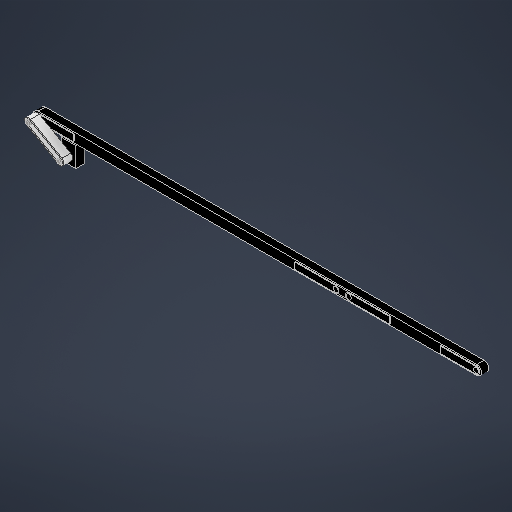
# Autodesk Inventor part: SACMI DPA MAIN CONVEYOR
Saved by Autodesk Inventor 2025 (Build 290162000, 162)
## iProperties
Created: 2024-05-26
Part Number: SACMI DPA MAIN CONVEYOR
Material: Generic
Document SubType Name: Modeling
Designer: zulet
Density: 1 g/cm^3
Appearance: Default
Author: zulet
Autodesk Inventor part; units mm, degrees
ref_plane "YZ Plane" through (0, 0, 0) normal (1, 0, 0) x (0, 1, 0)
ref_plane "XZ Plane" through (0, 0, 0) normal (0, 1, 0) x (-1, 0, 0)
ref_plane "XY Plane" through (0, 0, 0) normal (0, 0, 1) x (1, 0, 0)
sketch "Sketch1" plane through (0, 0, 0) normal (0, 0, 1) x (1, 0, 0)
  line L0 (-1550, 0) -> (1550, 0) construction
  line L1 (-1517, -33) -> (1517, -33)
  line L2 (1517, 33) -> (-1517, 33)
  arc A0 (-1517, 33) -> (-1517, -33) centre (-1517, 0) ccw
  arc A1 (1517, -33) -> (1517, 33) centre (1517, 0) ccw
  line L3 (-1517, 23) -> (1517, 23)
  arc A2 (1517, -23) -> (1517, 23) centre (1517, 0) ccw
  line L4 (1517, -23) -> (-1517, -23)
  arc A3 (-1517, 23) -> (-1517, -23) centre (-1517, 0) ccw
  line L5 (-1268, 23) -> (-1268, -23)
  line L6 (1268, 23) -> (1268, -23)
  circle A4 centre (1517, 0) radius 17.5
  circle A5 centre (-1517, 0) radius 17.5
  arc A6 (523, 0) -> (546, -23) centre (546, 0) ccw construction
  arc A7 (636, 23) -> (636, -23) centre (636, 0) ccw
  line L7 (264, 23) -> (264, -23)
  line L8 (918, 23) -> (918, -23)
  arc A8 (546, 23) -> (523, 0) centre (546, 0) ccw construction
  arc A9 (546, -23) -> (546, 23) centre (546, 0) ccw
  arc A10 (659, 0) -> (636, 23) centre (636, 0) ccw construction
  arc A11 (636, -23) -> (659, 0) centre (636, 0) ccw construction
  circle A12 centre (546, 0) radius 18
  circle A13 centre (636, 0) radius 18
  point P0 (0, 0)
  point P1 (0, 0)
  point P2 (-1550, 0)
  point P3 (1550, 0)
  dimension "d0" = 3100
  dimension "d1" = 66
  dimension "d2" = 10
  dimension "d3" = 282
  dimension "d4" = 282
  dimension "d5" = 35
  dimension "d6" = 35
  dimension "d7" = 282
  dimension "d8" = 282
  dimension "d9" = 90
  dimension "d10" = 350
  dimension "d45" = 5
  dimension "d46" = 5
  constraints: 24 point on circle, 20 end point, 18 point on line, 14 centre point, 8 tangent, 5 coincident, 4 perpendicular, 2 parallel, 1 horizontal, 1 midpoint, 3 other
  measures "d0" distance of L0.start L0.end
  measures "d1" diameter of A1
  measures "d2" distance between parallel lines of L2 L3
  measures "d3" distance from line of point (-1550, 0) L5
  measures "d4" distance from line of point (1550, 0) L6
  measures "d5" diameter of A4
  measures "d6" diameter of A5
  measures "d7" distance from line of L7 A6.centre
  measures "d8" distance from line of L8 A7.centre
  measures "d9" distance of A6.centre A7.centre
  measures "d10" distance between parallel lines of L6 L8
  measures "d45" radial gap between concentric circles of A9 A12
  measures "d46" radial gap between concentric circles of A13 A7
extrude "Extrusion1" add sketch "Sketch1" along normal mid plane 50 contours A0 L2 A1 L1
extrude "Extrusion2" add sketch "Sketch1" along normal mid plane 60 contours L3 L5 L4 A3 | L3 A9 L4 L7 | L3 L8 L4 A7 | L3 A2 L4 L6
extrude "Extrusion3" add sketch "Sketch1" along normal mid plane 50 contours L3 L7 L4 L5 | L3 L6 L4 L8
sketch "Sketch2" plane through (0, 0, 30) normal (0, 0, 1) x (1, 0, 0)
  circle A0 centre (-1517, 0) radius 17.5 projected
  line L0 (-1517, 0) -> (-1300.4936, -125) construction
  line L1 (-1530.75, -23.8157) -> (-1314.2436, -148.8157)
  line L2 (-1286.7436, -101.1843) -> (-1503.25, 23.8157)
  arc A1 (-1503.25, 23.8157) -> (-1530.75, -23.8157) centre (-1517, 0) ccw
  arc A2 (-1314.2436, -148.8157) -> (-1286.7436, -101.1843) centre (-1300.4936, -125) ccw
  line L3 (-1508.25, 15.1554) -> (-1291.7436, -109.8446)
  arc A3 (-1309.2436, -140.1554) -> (-1291.7436, -109.8446) centre (-1300.4936, -125) ccw
  line L4 (-1309.2436, -140.1554) -> (-1525.75, -15.1554)
  arc A4 (-1508.25, 15.1554) -> (-1525.75, -15.1554) centre (-1517, 0) ccw
  line L5 (-1517, -33) -> (1517, -33) projected
  line L6 (-1350.4936, -33) -> (-1250.4936, -33)
  line L7 (-1250.4936, -33) -> (-1250.4936, -175)
  line L8 (-1250.4936, -175) -> (-1350.4936, -175)
  line L9 (-1350.4936, -175) -> (-1350.4936, -33)
  circle A5 centre (-1300.4936, -125) radius 17.5
  line L10 (-1300.4936, -175) -> (-1300.4936, -33) construction
  point P0 (0, 0)
  point P1 (-1408.7468, -62.5)
  point P2 (-1250.4936, -33)
  point P3 (-1309.2436, -140.1554)
  point P4 (-1291.7436, -109.8446)
  point P5 (-1525.75, -15.1554)
  point P6 (-1508.25, 15.1554)
  dimension "d19" = 10
  dimension "d20" = 10
  dimension "d21" = 250
  dimension "d22" = 30
  dimension "d23" = 100
  dimension "d24" = 50
  constraints: 22 end point, 8 point on circle, 5 centre point, 5 tangent, 4 parallel, 3 midpoint, 2 point on line, 1 coincident, 1 horizontal, 1 perpendicular, 3 other
  measures "d19" radial gap between concentric circles of A1 A0
  measures "d20" distance between parallel lines of L2 L3
  measures "d21" distance of L0.start L0.end
  measures "d22" angle of L6 L0
  measures "d23" distance of L7.end L8.end
  measures "d24" distance from line of L8 L0.end
extrude "Extrusion4" add sketch "Sketch2" against normal blind 60 contours L9 L2 A2 L1 L4 A3 L3 | L3 A5 L4 L9 | L9 L5 L7 L8 L1 A2 L2
extrude "Extrusion5" add sketch "Sketch2" along normal blind 60 separate body contours A0 L4 L5 L1 A1 L2 L3 | L5 L2 L9 L3 | L4 L9 L1 L5 | L9 L2 A2 L1 L4 A3 L3
extrude "Extrusion6" add sketch "Sketch2" along normal blind 70 and the other way blind 10 contours A0 | A3 A5 bodies 1
chamfer "Chamfer2" distance 5 angle 45 2 edges at (-1534.5, 0, 100) (-1291.7436, -109.8446, 100)
chamfer "Chamfer3" distance 5 angle 45 2 edges at (-1300.4936, -33, -30) (-1300.4936, -33, 30)
chamfer "Chamfer4" distance 5 angle 45 6 edges at (-1250.4936, -33, 25) (-1250.4936, -33, 0) (-1250.4936, -33, -25.0001) (-1350.4936, -33, 25) (-1350.4936, -33, 0) (-1350.4936, -33, -25)
equation "\"d4\" = d3"
equation "\"d5\" = d6"
equation "\"d7\" = d3"
equation "\"d8\" = d3"
equation "\"d20\" = d19"
body "Solid1"
body "Solid2"
